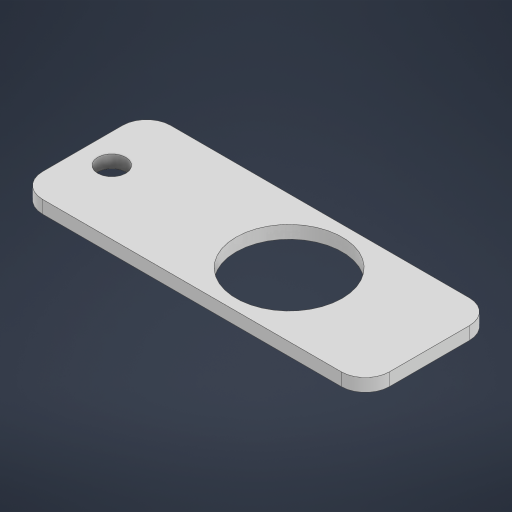
# Autodesk Inventor part: PCBAux
Saved by Autodesk Inventor 2023 (Build 270158000, 158)
## iProperties
Created: 2022-11-13
Part Number: PCBAux
Material: Generic
Document SubType Name: Modeling
Designer: jevan
Density: 1 g/cm^3
Appearance: Default
Author: jevan
Autodesk Inventor part; units mm, degrees
ref_plane "YZ Plane" through (0, 0, 0) normal (1, 0, 0) x (0, 1, 0)
ref_plane "XZ Plane" through (0, 0, 0) normal (0, 1, 0) x (-1, 0, 0)
ref_plane "XY Plane" through (0, 0, 0) normal (0, 0, 1) x (1, 0, 0)
sketch "Sketch1" plane through (0, 0, 0) normal (0, 1, 0) x (-1, 0, 0)
  line L0 (3, 0) -> (40.325, 0)
  line L1 (43.325, 3) -> (43.325, 13)
  line L2 (40.325, 16) -> (3, 16)
  line L3 (0, 13) -> (0, 3)
  circle A0 centre (17.525, 8) radius 6.625
  arc A1 (3, 16) -> (0, 13) centre (3, 13) ccw
  arc A2 (0, 3) -> (3, 0) centre (3, 3) ccw
  arc A3 (40.325, 0) -> (43.325, 3) centre (40.325, 3) ccw
  arc A4 (43.325, 13) -> (40.325, 16) centre (40.325, 13) ccw
  line L4 (10.9, 8) -> (17.525, 8)
  circle A5 centre (39.675, 8) radius 1.75
  point P0 (0, 0)
  point P1 (43.325, 16)
  point P2 (43.325, 0)
  point P3 (0, 16)
  dimension "d0" = 13.25
  dimension "d1" = 16
  dimension "d9" = 3
  dimension "d20" = 8
  dimension "d22" = 25.8
  dimension "d24" = 10.9
  dimension "d25" = 3.5
  dimension "d26" = 3.65
  constraints: 10 end point, 9 point on line, 8 point on circle, 8 tangent, 5 centre point, 3 equal radius, 2 coincident, 2 horizontal, 2 parallel, 1 horizontal alignment, 1 perpendicular, 2 other
  measures "d1" distance between parallel lines of L0 L2
  measures "d9" radius of A1
  measures "d20" distance from line of L2 point (17.525, 8)
  measures "d22" distance from line of L1 point (17.525, 8)
  measures "d24" distance from line of L3 L4.start
  measures "d25" diameter of A5
  measures "d26" distance from line of L1 A5.centre
extrude "Extrusion1" add sketch "Sketch1" along normal blind 1.6
body "Solid1"
